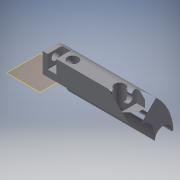
# Autodesk Inventor part: 24_Klammer_rechts
Saved by Autodesk Inventor 2016 (Build 200138000, 138)
## iProperties
Created: 2016-10-24
Part Number: 24_Klammer_rechts
Material: Generisch
Document SubType Name: Modeling
Designer: Bene
Density: 1 g/cm^3
Appearance: Vorgabe
Author: Bene
Autodesk Inventor part; units mm, degrees
ref_plane "YZ Plane" through (0, 0, 0) normal (1, 0, 0) x (0, 1, 0)
ref_plane "XZ Plane" through (0, 0, 0) normal (0, 1, 0) x (-1, 0, 0)
ref_plane "Arbeitsebene1" through (0, 0, 15) normal (0, 0, 1) x (1, 0, 0)
sketch "Skizze1" plane through (0, 0, 15) normal (0, 0, 1) x (1, 0, 0)
  circle A0 centre (15, 4.6239) radius 3 construction
  line L0 (15, 4.6239) -> (43, 4.6239) construction
  line L1 (1.5, 0.1239) -> (56.5, 0.1239)
  line L2 (56.5, 0.1239) -> (56.5, 9.1239)
  line L3 (56.5, 9.1239) -> (1.5, 9.1239)
  line L4 (1.5, 9.1239) -> (1.5, 0.1239)
  line L5 (1.5, 0.1239) -> (56.5, 9.1239) construction
  line L6 (56.5, 0.1239) -> (1.5, 9.1239) construction
  circle A1 centre (15, 4.6239) radius 3.15
  circle A2 centre (43, 4.6239) radius 3.15
  point P0 (0, 0)
  point P1 (29, 4.6239)
  dimension "d1" = 55
  dimension "d2" = 9
  dimension "d3" = 6.3
  dimension "d4" = 6.3
  constraints: 14 end point, 3 midpoint, 2 centre point, 2 coincident, 2 horizontal, 2 parallel, 1 perpendicular
  measures "d1" distance of L3.end L2.end
  measures "d2" distance of L2.end L1.end
  measures "d3" diameter of A1
  measures "d4" diameter of A2
extrude "Extrusion1" add sketch "Skizze1" along normal blind 5
sketch "Skizze2" plane through (0, 0, 20) normal (0, 0, 1) x (1, 0, 0)
  circle A0 centre (43, 4.6239) radius 3.15 projected
  circle A1 centre (15, 4.6239) radius 3.15 projected
  line L0 (1.5, 0.1239) -> (56.5, 0.1239) projected
  line L1 (56.5, 0.1239) -> (56.5, 9.1239) projected
  line L2 (56.5, 9.1239) -> (1.5, 9.1239) projected
  line L3 (1.5, 9.1239) -> (1.5, 0.1239) projected
  line L4 (56.5, 9.1239) -> (1.5, 9.1239) projected
  line L5 (1.5, 0.1239) -> (56.5, 0.1239) projected
  line L6 (1.5, 9.1239) -> (19.5, 9.1239)
  line L7 (19.5, 9.1239) -> (19.5, 0.1239)
  line L8 (19.5, 0.1239) -> (1.5, 0.1239)
  line L9 (1.5, 0.1239) -> (1.5, 9.1239)
  line L10 (56.5, 9.1239) -> (38.5, 9.1239)
  line L11 (38.5, 9.1239) -> (38.5, 0.1239)
  line L12 (38.5, 0.1239) -> (56.5, 0.1239)
  line L13 (56.5, 0.1239) -> (56.5, 9.1239)
  point P0 (0, 0)
  dimension "d7" = 18
  dimension "d8" = 18
  constraints: 16 end point, 4 parallel, 2 horizontal, 2 perpendicular, 2 point on line
  measures "d7" distance of L7.end L8.end
  measures "d8" distance of L12.end L11.end
extrude "Extrusion2" add sketch "Skizze2" along normal blind 7
sketch "Skizze3" plane through (1.5, 0.1239, 15) normal (-1, 0, 0) x (0, 0, 1)
  line L0 (5, 9) -> (5, 0) projected
  line L1 (0, 9) -> (0, 0) projected
  line L2 (0, 0) -> (12, 0) projected
  line L3 (12, 9) -> (12, 0) projected
  line L4 (0, 9) -> (12, 9) projected
  circle A0 centre (8.5, 4.5) radius 2.25
  point P0 (-15, -0.1239)
  dimension "d11" = 4.5
  dimension "d12" = 4.5
  dimension "d13" = 3.5
  constraints: 1 centre point
  measures "d11" diameter of A0
  measures "d12" distance from line of A0.centre L4
  measures "d13" distance from line of A0.centre L3
extrude "Extrusion3" cut sketch "Skizze3" against normal blind 12 contours A0
sketch "Skizze4" plane through (56.5, 0.1239, 15) normal (1, 0, 0) x (0, 0, -1)
  spline S0 degree 2 poles (-10.75, 4.5) (-10.75, 8.3971) (-7.375, 6.4486) (-4, 4.5) (-7.375, 2.5514) (-10.75, 0.6029) (-10.75, 4.5) knots 0 0 0 0.333333 0.333333 0.666667 0.666667 1 1 1 weights 1 0.5 1 0.5 1 0.5 1 projected
  point P0 (15, -0.1239)
  constraints: 1 other
extrude "Extrusion4" cut sketch "Skizze4" against normal blind 12
sketch "Skizze6" plane through (0, 0, 27) normal (0, 0, 1) x (1, 0, 0)
  circle A0 centre (15, 4.6239) radius 3.15 projected
  circle A1 centre (43, 4.6239) radius 3.15 projected
  line L0 (56.5, 0.1239) -> (56.5, 9.1239) projected
  line L1 (1.5, 9.1239) -> (1.5, 0.1239) projected
  line L2 (1.5, 0.1239) -> (56.5, 0.1239) projected
  line L3 (1.5, 6.8739) -> (12.7955, 6.8739) construction
  line L4 (1.5, 2.3739) -> (12.7955, 2.3739) construction
  line L5 (56.5, 6.8739) -> (45.2045, 6.8739) construction
  line L6 (56.2124, 3.2478) -> (53, 3.2478) construction
  line L7 (1.5, 0.1239) -> (56.5, 0.1239) construction
  line L8 (56.5, 9.1239) -> (1.5, 9.1239) construction
  line L9 (4.5, 0.1239) -> (9.5, 0.1239) construction
  line L10 (9.5, 0.1239) -> (9.5, 9.1239) construction
  line L11 (9.5, 9.1239) -> (4.5, 9.1239) construction
  line L12 (4.5, 9.1239) -> (4.5, 0.1239) construction
  line L13 (4.5, 0.1239) -> (9.5, 0.1239)
  line L14 (9.5, 0.1239) -> (9.5, 9.1239)
  line L15 (9.5, 9.1239) -> (4.5, 9.1239)
  line L16 (4.5, 9.1239) -> (4.5, 0.1239)
  line L17 (48.5, 0.1239) -> (53.5, 0.1239)
  line L18 (53.5, 0.1239) -> (53.5, 9.1239)
  line L19 (53.5, 9.1239) -> (48.5, 9.1239)
  line L20 (48.5, 9.1239) -> (48.5, 0.1239)
  line L21 (56.5, 9.1239) -> (1.5, 9.1239) projected
  point P0 (0, 0)
  point P1 (38.5, 9.1239)
  point P2 (38.5, 0.1239)
  point P3 (19.5, 0.1239)
  point P4 (19.5, 9.1239)
  point P5 (49.7876, 3.2478)
  dimension "d23" = 5
  dimension "d24" = 5
  dimension "d27" = 3
  dimension "d28" = 3
  constraints: 24 end point, 6 parallel, 4 point on line, 3 horizontal, 3 perpendicular, 2 other
  measures "d23" distance of L11.end L10.end
  measures "d24" distance of L19.end L18.end
  measures "d27" distance between parallel lines of L18 L0
  measures "d28" distance between parallel lines of L1 L12
extrude "Extrusion6" cut sketch "Skizze6" against normal blind 8 contours L2 L20 L19 L18 | L2 L16 L15 L14
sketch "Skizze7" plane through (1.5, 0.1239, 15) normal (-1, 0, 0) x (0, 0, 1)
  circle A0 centre (8.5, 4.5) radius 2.25 projected
  line L0 (0, 9) -> (0, 0) projected
  line L1 (0, 0) -> (12, 0) projected
  line L2 (12, 9) -> (12, 0) projected
  line L3 (0, 9) -> (12, 9) projected
  arc A1 (-12.9416, 12) -> (-12.9416, 22) centre (-12.5523, 17) ccw
  line L4 (-12.9416, 22) -> (-12.9416, 12) construction
  line L5 (-12.9416, 22) -> (-2.9416, 22) construction
  arc A2 (0, 9) -> (-12.9416, 12) centre (-16.3892, -32.2866) ccw
  line L6 (12, 0) -> (12, 9) projected
  line L7 (-12.9416, 22) -> (-12.9416, 23)
  line L8 (-12.9416, 22) -> (-11.9416, 22) construction
  arc A3 (12, 9) -> (-12.9416, 23) centre (-14.7562, -9.45) ccw
  point P0 (-15, -0.1239)
  dimension "d29" = 10
  dimension "d30" = 90
  dimension "d34" = 1
  dimension "d35" = 90
  dimension "d37" = 3
  constraints: 8 end point, 6 point on circle, 3 centre point, 2 horizontal, 2 perpendicular, 1 tangent, 1 vertical
  measures "d29" distance of L4.start L4.end
  measures "d30" angle of L4 L5
  measures "d34" distance of L4.start L7.end
  measures "d35" angle of L8 L7
  measures "d37" distance from line of L4.end L3
extrude "Extrusion7" add sketch "Skizze7" against normal up to surface (55 mm away) contours A2 A1 L7 A3 L3
fillet "Rundung2" radius 8 1 edges at (29, 9.1239, 15)
fillet "Rundung3" radius 8 1 edges at (29, 9.1239, 27)
